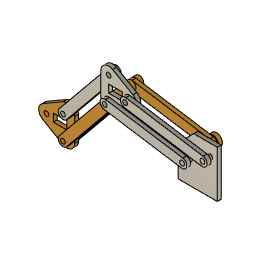
Basic Robot 4 bar v2 Lab v1 (Autodesk Fusion 360 design; units mm, degrees)
Autodesk Fusion 360 part; units mm, degrees
note: some values were not read from the file. Set by a fixed rule: which sketch regions a step uses.
sketch "Sketch1" plane through (0, 0, 0) normal (0, 1, 0) x (1, 0, 0) in component "Component"
  line L0 (0, 0) -> (50, 0)
  line L1 (50, 0) -> (50, -60)
  line L2 (50, -60) -> (0, -60)
  line L3 (0, -60) -> (0, 0)
  dimension "d1" = 50
  dimension "d2" = 60
  constraint horizontal L0
  constraint vertical L1
  constraint horizontal L2
  constraint vertical L3
  constraint coincident L0.start L3.end
  measures "d1" distance of L0.start L0.end
  measures "d2" distance of L0.start L2.end
extrude "Extrude1" add sketch "Sketch1" along normal blind 5 makes body 1 in component "Component"
sketch "Sketch1 (2)" plane through (0, 0, 0) normal (0, 1, 0) x (1, 0, 0) in component "Component'"
  line L0 (0, -6) -> (100, -6)
  arc A0 (100, -6) -> (100, 6) centre (100, 0) ccw
  line L1 (100, 6) -> (0, 6)
  arc A1 (0, 6) -> (0, -6) centre (0, 0) ccw
  line L2 (0, 0) -> (100, 0) construction
  circle A2 centre (0, 0) radius 3
  circle A3 centre (100, 0) radius 3
  dimension "d8" = 12
  dimension "d9" = 6
  dimension "d10" = 6
  dimension "d13" = 100
  constraint tangent L0 A0
  constraint tangent A0 L1
  constraint parallel L0 L1
  constraint tangent L1 A1
  constraint tangent L0 A1
  constraint horizontal L2
  constraint coincident A1.centre L2.start
  constraint concentric A0 A3
  measures "d8" diameter of A0
  measures "d9" diameter of A2
  measures "d10" diameter of A3
  measures "d13" distance of A1.centre A0.centre
extrude "Extrude1'" add sketch "Sketch1 (2)" along normal blind 5 separate body makes body 2 in component "Component'"
sketch "Sketch1 (3)" plane through (0, 0, 0) normal (0, 1, 0) x (1, 0, 0) in component "Component''"
  line L0 (0, -6) -> (130, -6)
  arc A0 (130, -6) -> (130, 6) centre (130, 0) ccw
  line L1 (130, 6) -> (0, 6)
  arc A1 (0, 6) -> (0, -6) centre (0, 0) ccw
  line L2 (0, 0) -> (130, 0) construction
  circle A2 centre (0, 0) radius 3
  circle A3 centre (30, 0) radius 3
  circle A4 centre (130, 0) radius 3
  dimension "d14" = 12
  dimension "d15" = 6
  dimension "d16" = 6
  dimension "d17" = 6
  dimension "d18" = 30
  dimension "d19" = 100
  constraint tangent L0 A0
  constraint tangent A0 L1
  constraint parallel L0 L1
  constraint tangent L1 A1
  constraint tangent L0 A1
  constraint horizontal L2
  constraint coincident A1.centre L2.start
  constraint coincident L2 A3.centre
  constraint concentric A0 A4
  measures "d14" diameter of A0
  measures "d15" diameter of A2
  measures "d16" diameter of A3
  measures "d17" diameter of A4
  measures "d18" distance of A1.centre A3.centre
  measures "d19" distance of A3.centre A0.centre
extrude "Extrude1''" add sketch "Sketch1 (3)" along normal blind 5 separate body makes body 3 in component "Component''"
sketch "Sketch1 (4)" plane through (0, 0, 0) normal (0, 1, 0) x (1, 0, 0) in component "Component'''"
  line L0 (0, -7.5) -> (30, -7.5)
  arc A0 (30, -7.5) -> (30, 7.5) centre (30, 0) ccw
  line L1 (30, 7.5) -> (0, 7.5)
  arc A1 (0, 7.5) -> (0, -7.5) centre (0, 0) ccw
  line L2 (0, 0) -> (30, 0) construction
  circle A2 centre (0, 0) radius 3
  circle A3 centre (30, 0) radius 3
  dimension "d8_1" = 15
  dimension "d9_1" = 6
  dimension "d10_1" = 6
  dimension "d13_1" = 30
  constraint tangent L0 A0
  constraint tangent A0 L1
  constraint parallel L0 L1
  constraint tangent L1 A1
  constraint tangent L0 A1
  constraint horizontal L2
  constraint coincident A1.centre L2.start
  constraint concentric A0 A3
  measures "d8_1" diameter of A0
  measures "d9_1" diameter of A2
  measures "d10_1" diameter of A3
  measures "d13_1" distance of A1.centre A0.centre
extrude "Extrude1'''" add sketch "Sketch1 (4)" along normal blind 5 separate body makes body 4 in component "Component'''"
sketch "Sketch1 (5)" plane through (0, 0, 0) normal (0, 1, 0) x (1, 0, 0) in component "Component''''"
  circle A0 centre (0, 0) radius 3
  line L0 (0, 0) -> (-30, 0) construction
  line L1 (-30, 0) -> (-15, -25.9808) construction
  line L2 (-15, -25.9808) -> (0, 0) construction
  line L3 (17.3205, 10) -> (-47.3205, 10)
  line L4 (-47.3205, 10) -> (-15, -45.9808)
  line L5 (-15, -45.9808) -> (17.3205, 10)
  circle A1 centre (-15, -25.9808) radius 3
  circle A2 centre (-30, 0) radius 3
  line L6 (-20, -17.3205) -> (-10, -17.3205)
  line L7 (-10, -17.3205) -> (-10, 0)
  line L8 (-10, 0) -> (-20, 0)
  line L9 (-20, 0) -> (-20, -17.3205)
  dimension "d126" = 30
  dimension "d127" = 10
  dimension "d128" = 6
  dimension "d375" = 10
  constraint coincident A0.centre L0.start
  constraint horizontal L0
  constraint equal L1 L2
  constraint equal L0 L2
  constraint coincident L1.end L2.start
  constraint coincident L0.end L1.start
  constraint equal A1 A2
  constraint equal A0 A1
  constraint horizontal L6
  constraint vertical L7
  constraint horizontal L8
  constraint vertical L9
  constraint coincident L0 L7.end
  constraint coincident L1 L6.start
  constraint coincident L2 L6.end
  measures "d126" distance of A0.centre L0.end
  measures "d128" diameter of A0
  measures "d375" distance of L6.start L6.end
extrude "Extrude1''''" add sketch "Sketch1 (5)" along normal blind 5 separate body makes body 5 in component "Component''''"
fillet "Fillet1" radius 10 3 edges at (-15, 2.5, 45.9808) (17.3205, 2.5, -10) (-47.3205, 2.5, -10) on bodies 5 in component "Component''''"
sketch "Sketch2" plane through (0, 5, 0) normal (0, 1, 0) x (-1, 0, 0) in component "Component"
  line L0 (0, 60) -> (-50, 60)
  line L1 (-50, 60) -> (-50, 0)
  line L2 (-50, 0) -> (0, 0)
  line L3 (0, 0) -> (0, 60)
  circle A0 centre (-35, 30) radius 3
  dimension "d202" = 6
  dimension "d203" = 15
  dimension "d204" = 30
  measures "d202" diameter of A0
  measures "d203" distance of L1 A0.centre
  measures "d204" distance of L2 A0.centre
extrude "Extrude2" add sketch "Sketch2" along normal blind 10 and the other way blind 15 contours A0 bodies 1 in component "Component"
sketch "Sketch3" plane through (0, 5, 0) normal (0, 1, 0) x (-1, 0, 0) in component "Component"
  circle A0 centre (-35, 30) radius 3
  line L0 (0, 60) -> (-50, 60)
  line L1 (-50, 60) -> (-50, 0)
  line L2 (-50, 0) -> (0, 0)
  line L3 (0, 0) -> (0, 60)
  circle A1 centre (-9.0192, 45) radius 3
  line L4 (-35, 30) -> (-9.0192, 45) construction
  line L5 (-35, 30) -> (-5, 30) construction
  dimension "d216" = 6
  dimension "d217" = 30
  dimension "d218" = 30
  constraint horizontal L5
  constraint coincident A0.centre L4.start
  constraint coincident A1.centre L4.end
  measures "d216" diameter of A1
  measures "d217" angle of L4 L5
  measures "d218" distance of A0.centre A1.centre
chamfer "Chamfer2" distance 20 angle 45 1 edges at (50, 2.5, 60) on bodies 1 in component "Component"
extrude "Extrude4" add sketch "Sketch3" along normal blind 10 contours A1 bodies 1 in component "Component"
component "Component" placed x (1, 0, 0) y (0, 1, 0) z (0, 0, 1) at (0, 0, 0)
component "Component'" placed x (0.318151, 0, 0.94804) y (0, 1, 0) z (-0.94804, 0, 0.318151) at (12.4337, 81.0919, 126.0474)
component "Component''" placed x (0.771336, 0, 0.636429) y (0, 1, 0) z (-0.636429, 0, 0.771336) at (11.8599, -10, 110.9071)
component "Component'''" placed x (-0.771336, 0, -0.636429) y (0, 1, 0) z (0.636429, 0, -0.771336) at (35, -10, 30)
component "Component'" placed x (0, 0, 1) y (0, 1, 0) z (-1, 0, 0) at (11.8599, -5, 10.9071)
component "Component''''" placed x (0.496725, 0, -0.867908) y (0, 1, 0) z (0.867908, 0, 0.496725) at (112.1336, -5, 193.6429)
component "Component''''" placed x (0.289419, 0, 0.957202) y (0, 1, 0) z (-0.957202, 0, 0.289419) at (43.6826, 5, 158.7161)
component "Component'" placed x (0.318151, 0, 0.94804) y (0, 1, 0) z (-0.94804, 0, 0.318151) at (-43.9483, 75.8536, 128.0566)
component "Component'" placed x (0.806145, 0, -0.591717) y (0, 1, 0) z (0.591717, 0, 0.806145) at (48.7488, 36.7536, 212.9086)
component "Component'" placed x (0.025787, 0, 0.999667) y (0, 1, 0) z (-0.999667, 0, 0.025787) at (35, -5, 30)
component "Component''" placed x (0.771336, 0, 0.636429) y (0, 1, 0) z (-0.636429, 0, 0.771336) at (11.8599, 0, 110.9071)
